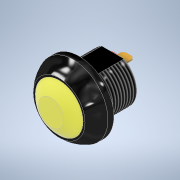
# Autodesk Inventor part: Sprung Button DigiKey EG9580-ND
Saved by Autodesk Inventor 2021 (Build 250183000, 183)
## iProperties
Created: 2020-07-20
Part Number: Sprung Button DigiKey EG9580-ND
Material: Generic
Document SubType Name: Modeling
Designer: jgray
Density: 1 g/cm^3
Appearance: Anodized - Black
Author: jgray
Autodesk Inventor part; units mm, degrees
ref_plane "YZ Plane" through (0, 0, 0) normal (1, 0, 0) x (0, 1, 0)
ref_plane "XZ Plane" through (0, 0, 0) normal (0, 1, 0) x (-1, 0, 0)
ref_plane "XY Plane" through (0, 0, 0) normal (0, 0, 1) x (1, 0, 0)
sketch "Sketch1" plane through (0, 0, 0) normal (0, 1, 0) x (-1, 0, 0)
  line L0 (-8.75, -0.75) -> (8.75, -0.75)
  line L1 (8.75, -0.75) -> (8.75, 0.75)
  line L2 (8.75, 0.75) -> (-8.75, 0.75)
  line L3 (-8.75, 0.75) -> (-8.75, -0.75)
  line L4 (-8.75, -0.75) -> (8.75, 0.75) construction
  line L5 (8.75, -0.75) -> (-8.75, 0.75) construction
  line L6 (6.5, 4.25) -> (-6.5, 4.25)
  line L7 (0, 21.8262) -> (0, -10.0956)
  arc A0 (-6.5, 4.25) -> (-8.75, 0.75) centre (0, -2.4018) ccw
  arc A1 (8.75, 0.75) -> (6.5, 4.25) centre (0, -2.4018) ccw
  line L8 (3.2, 6.25) -> (-3.2, 6.25)
  line L9 (6, 4.25) -> (-6, 4.25)
  arc A2 (6, 4.25) -> (3.2, 6.25) centre (0, -1.19) ccw
  arc A3 (7.8812, 0.6755) -> (7.8632, 0.75) centre (0, -1.19) ccw
  arc A4 (8.087, -0.75) -> (8.0837, -0.6929) centre (0, -1.19) ccw
  arc A5 (-8.0837, -0.6929) -> (-8.087, -0.75) centre (0, -1.19) ccw
  arc A6 (-3.2, 6.25) -> (-6, 4.25) centre (0, -1.19) ccw
  arc A7 (-7.8632, 0.75) -> (-7.8812, 0.6755) centre (0, -1.19) ccw
  line L10 (-6, -9.25) -> (6, -9.25)
  line L11 (6, -9.25) -> (6, -0.75)
  line L12 (6, -0.75) -> (-6, -0.75)
  line L13 (-6, -0.75) -> (-6, -9.25)
  line L14 (-6, -9.25) -> (6, -0.75) construction
  line L15 (6, -9.25) -> (-6, -0.75) construction
  line L16 (-5, -9.75) -> (5, -9.75)
  line L17 (5, -9.75) -> (5, -9.25)
  line L18 (5, -9.25) -> (-5, -9.25)
  line L19 (-5, -9.25) -> (-5, -9.75)
  line L20 (-5, -9.75) -> (5, -9.25) construction
  line L21 (5, -9.75) -> (-5, -9.25) construction
  point P0 (0, 0)
  point P1 (0, 4.25)
  point P2 (0, 0)
  point P3 (0, 6.25)
  point P4 (0, 4.25)
  point P5 (0, -5)
  point P6 (0, -9.5)
  point P7 (0, -9.75)
  dimension "d0" = 17.5
  dimension "d1" = 1.5
  dimension "d2" = 13
  dimension "d3" = 5
  dimension "d4" = 2
  dimension "d5" = 6.4
  dimension "d6" = 12
  dimension "d7" = 12
  dimension "d8" = 8.5
  dimension "d9" = 10
  dimension "d10" = 0.5
  constraints: 42 end point, 16 point on circle, 10 midpoint, 10 point on line, 8 centre point, 6 parallel, 5 horizontal, 3 perpendicular, 2 collinear, 11 other
  measures "d0" distance of L2.end L1.end
  measures "d1" distance of L0.end L1.end
  measures "d2" distance of L6.end L6.start
  measures "d3" distance between parallel lines of L0 L6
  measures "d4" distance between parallel lines of L6 L8
  measures "d5" distance of L8.end L8.start
  measures "d6" distance of L9.start L9.end
  measures "d7" distance of L12.end L11.end
  measures "d8" distance of L11.end L10.end
  measures "d9" distance of L18.end L17.end
  measures "d10" distance of L17.end L16.end
revolve "Revolution1" add sketch "Sketch1" angle 360 about axis through (0, 0, 21.8262) along (0, 0, -1) contours L3 L2 L7 L0 | A0 L6 L7 L2 | L0 L7 L10 L13 | A6 L8 L7 L6 | L7 L16 L19 L10
sketch "Sketch2" plane through (0, 0, -9.75) normal (0, 0, -1) x (-1, 0, 0)
  line L0 (0, -14.0708) -> (0, 14.0708) construction
  line L1 (1.4, -2.94) -> (-1.4, -2.94)
  line L2 (-1.4, -2.94) -> (-1.4, -2.54)
  line L3 (-1.4, -2.54) -> (1.4, -2.54)
  line L4 (1.4, -2.54) -> (1.4, -2.94)
  line L5 (1.4, -2.94) -> (-1.4, -2.54) construction
  line L6 (-1.4, -2.94) -> (1.4, -2.54) construction
  line L7 (1.4, 2.94) -> (-1.4, 2.94)
  line L8 (-1.4, 2.94) -> (-1.4, 2.54)
  line L9 (-1.4, 2.54) -> (1.4, 2.54)
  line L10 (1.4, 2.54) -> (1.4, 2.94)
  line L11 (1.4, 2.94) -> (-1.4, 2.54) construction
  line L12 (-1.4, 2.94) -> (1.4, 2.54) construction
  point P0 (0, 0)
  point P1 (0, 0)
  point P2 (0, -2.74)
  point P3 (0, 2.74)
  dimension "d12" = 2.8
  dimension "d13" = 0.4
  dimension "d14" = 2.8
  dimension "d15" = 0.4
  dimension "d16" = 5.08
  dimension "d17" = 2.54
  constraints: 26 end point, 5 midpoint, 4 parallel, 2 horizontal, 2 perpendicular, 2 point on line, 1 coincident, 1 vertical
  measures "d12" distance of L2.end L3.end
  measures "d13" distance of L1.end L2.end
  measures "d14" distance of L9.end L8.end
  measures "d15" distance of L8.end L7.end
  measures "d16" distance between parallel lines of L9 L3
  measures "d17" distance from line of point (0, 0) L3
extrude "Extrusion1" add sketch "Sketch2" along normal blind 3.5
chamfer "Chamfer1" distance 0.5 angle 45 4 edges at (1.4, -2.74, -13.25) (-1.4, -2.74, -13.25) (1.4, 2.74, -13.25) (-1.4, 2.74, -13.25)
thread "Thread1" size "M12x0.75" class "6g" standard "ANSI Metric M Profile" length 12.5
sketch "Sketch3" plane through (0, 0, -9.25) normal (0, 0, -1) x (-1, 0, 0)
  line L0 (12.7626, -5.3) -> (-12.9759, -5.3)
  line L1 (12.7626, 5.3) -> (-13.4328, 5.3)
  line L2 (14.0115, 0) -> (-13.4328, 0) construction
  circle A0 centre (0, 0) radius 6 construction
  circle A1 centre (0, 0) radius 6
  point P0 (0, 0)
  point P1 (-2.8125, 5.3)
  point P2 (2.8125, 5.3)
  point P3 (-2.8125, -5.3)
  point P4 (2.8125, -5.3)
  dimension "d25" = 10.6
  constraints: 6 end point, 3 horizontal, 1 centre point, 1 coincident, 1 point on line, 1 other
  measures "d25" distance between parallel lines of L1 L0
extrude "Extrusion2" cut sketch "Sketch3" against normal up to surface (8.5 mm away) contours A1 L0 | A1 L1
body "Solid1"
